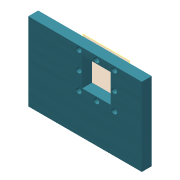
# Autodesk Inventor part: cellSTORM_Base_v0
Saved by Autodesk Inventor 2019 (Build 230136000, 136)
## iProperties
Created: 2019-10-29
Part Number: cellSTORM_Base_v0
Material: Generic
Document SubType Name: Modeling
Designer: diederichbenedict
Density: 1 g/cm^3
Appearance: Cadet Blue
Author: diederichbenedict
Autodesk Inventor part; units mm, degrees
ref_plane "YZ Plane" through (0, 0, 0) normal (1, 0, 0) x (0, 1, 0)
ref_plane "XZ Plane" through (0, 0, 0) normal (0, 1, 0) x (-1, 0, 0)
ref_plane "XY Plane" through (0, 0, 0) normal (0, 0, 1) x (1, 0, 0)
ref_plane "Work Plane1" through (0, 0, 0) normal (0, 0, 1) x (1, 0, 0)
sketch "Sketch1" plane through (0, 0, 0) normal (0, 0, 1) x (1, 0, 0)
  circle A0 centre (0, 25) radius 1.95 construction
  circle A1 centre (-25, 0) radius 1.95 construction
  circle A2 centre (-25, -25) radius 1.95 construction
  circle A3 centre (25, 25) radius 1.95 construction
  circle A4 centre (25, -25) radius 1.95 construction
  circle A5 centre (-25, 25) radius 1.95 construction
  circle A6 centre (25, 0) radius 1.95 construction
  circle A7 centre (0, -25) radius 1.95 construction
  line L0 (-28, 30) -> (-30, 28) construction
  line L1 (-30, 28) -> (-30, -28) construction
  line L2 (-30, -28) -> (-28, -30) construction
  line L3 (-28, -30) -> (28, -30) construction
  line L4 (28, -30) -> (30, -28) construction
  line L5 (30, -28) -> (30, 28) construction
  line L6 (30, 28) -> (28, 30) construction
  line L7 (28, 30) -> (-28, 30) construction
  circle A8 centre (35, -56) radius 1 construction
  circle A9 centre (5, -48.5) radius 1 construction
  circle A10 centre (5, -64.5) radius 1.0474 construction
  circle A11 centre (-5, -64.5) radius 1 construction
  circle A12 centre (-5, -56) radius 1 construction
  circle A13 centre (-5, -48.5) radius 1 construction
  circle A14 centre (5, -56) radius 1 construction
  circle A15 centre (35, -48) radius 1 construction
  circle A16 centre (35, -64) radius 1 construction
  line L8 (38, -40) -> (38, -72) construction
  line L9 (38, -40) -> (-10, -40) construction
  line L10 (-10, -72) -> (-10, -40) construction
  line L11 (38, -72) -> (-10, -72) construction
  line L12 (38, -71) -> (38, -41) construction
  line L13 (38, -71) -> (48, -71) construction
  line L14 (48, -41) -> (48, -71) construction
  line L15 (38, -41) -> (48, -41) construction
  line L16 (56, -75) -> (-52.5, -75)
  line L17 (-52.5, -75) -> (-52.5, -30)
  line L18 (-52.5, -30) -> (56, -30)
  line L19 (56, -30) -> (56, -75)
  line L20 (-40, -41.1445) -> (-40, -68) construction
  line L21 (-41, -39.0927) -> (-41, -47.7587) construction
  line L22 (-41, -39.0927) -> (-46.5, -39.0927) construction
  line L23 (-46.5, -47.7587) -> (-46.5, -39.0927) construction
  line L24 (-41, -47.7587) -> (-46.5, -47.7587) construction
  line L25 (-41, -60.5) -> (-41, -64) construction
  line L26 (-41, -60.5) -> (-46.5, -60.5) construction
  line L27 (-46.5, -64) -> (-46.5, -60.5) construction
  line L28 (-41, -64) -> (-46.5, -64) construction
  line L29 (64, 30) -> (-96, 30)
  line L30 (-96, 30) -> (-96, -80)
  line L31 (-96, -80) -> (64, -80)
  line L32 (64, -80) -> (64, 30)
  line L33 (20, -20) -> (-20, -20)
  line L34 (-20, -20) -> (-20, 20)
  line L35 (-20, 20) -> (20, 20)
  line L36 (20, 20) -> (20, -20)
  line L37 (20, -20) -> (-20, 20) construction
  line L38 (-20, -20) -> (20, 20) construction
  line L39 (-52.5, -30) -> (-30, -30)
  line L40 (-30, -30) -> (-30, -25)
  line L41 (-30, -25) -> (-52.5, -25)
  line L42 (-52.5, -25) -> (-52.5, -30)
  point P0 (0, 0)
  dimension "d1" = 3
  dimension "d2" = 8
  dimension "d4" = 6
  dimension "d5" = 160
  dimension "d6" = 110
  dimension "d7" = 8
  dimension "d19" = 40
  dimension "d20" = 40
  dimension "d28" = 5
  dimension "d29" = 0
  constraints: 36 end point, 8 parallel, 4 horizontal, 4 perpendicular, 2 midpoint, 1 point on line
  measures "d1" distance between parallel lines of L11 L16
  measures "d2" distance between parallel lines of L19 L14
  measures "d4" distance between parallel lines of L27 L17
  measures "d5" distance of L31.end L30.end
  measures "d6" distance of L30.end L29.end
  measures "d7" distance between parallel lines of L32 L19
  measures "d19" distance of L34.end L35.end
  measures "d20" distance of L33.end L34.end
  measures "d28" distance of L40.end L39.end
  measures "d29" distance between parallel lines of L18 L3
extrude "Extrusion1" add sketch "Sketch1" along normal blind 10
sketch "Sketch2" plane through (0, 0, 10) normal (0, 0, 1) x (1, 0, 0)
  line L0 (-30, -30) -> (56, -30) projected
  line L1 (56, -30) -> (56, -75) projected
  line L2 (56, -75) -> (-52.5, -75) projected
  line L3 (64, 30) -> (-96, 30) projected
  line L4 (-96, 30) -> (-96, -80) projected
  line L5 (-96, -80) -> (64, -80) projected
  line L6 (64, -80) -> (64, 30) projected
  line L7 (20, -20) -> (20, 20) projected
  line L8 (-20, -20) -> (20, -20)
  line L9 (20, -20) -> (20, 20)
  line L10 (20, 20) -> (-20, 20)
  line L11 (-20, 20) -> (-20, -20)
  line L12 (-20, -20) -> (20, 20) construction
  line L13 (20, -20) -> (-20, 20) construction
  line L14 (-52.5, -25) -> (-30, -25) projected
  line L15 (-30, -25) -> (-30, -30) projected
  line L16 (-52.5, -75) -> (-52.5, -25) projected
  point P0 (0, 0)
  constraints: 12 end point, 2 midpoint, 2 parallel, 1 horizontal, 1 perpendicular
extrude "Extrusion2" add sketch "Sketch2" along normal blind 4 contours L0 L1 L2 L16 L14 L15 | L6 L5 L4 L3
sketch "Sketch3" plane through (0, 0, 14) normal (0, 0, 1) x (1, 0, 0)
  circle A0 centre (0, 25) radius 1.95 construction
  circle A1 centre (-25, 0) radius 1.95 construction
  circle A2 centre (-25, -25) radius 1.95 construction
  circle A3 centre (25, 25) radius 1.95 construction
  circle A4 centre (25, -25) radius 1.95 construction
  circle A5 centre (-25, 25) radius 1.95 construction
  circle A6 centre (25, 0) radius 1.95 construction
  circle A7 centre (0, -25) radius 1.95 construction
  line L0 (-28, 30) -> (-30, 28) construction
  line L1 (-30, 28) -> (-30, -28) construction
  line L2 (-30, -28) -> (-28, -30) construction
  line L3 (-28, -30) -> (28, -30) construction
  line L4 (28, -30) -> (30, -28) construction
  line L5 (30, -28) -> (30, 28) construction
  line L6 (30, 28) -> (28, 30) construction
  line L7 (28, 30) -> (-28, 30) construction
  point P0 (0, 0)
hole "Hole1" at (25, 25, 14) at (0, 25, 14) at (-25, 25, 14) at (-25, 0, 14) at (-25, -25, 14) at (0, -25, 14) at (25, -25, 14) at (25, 0, 14) direction (0, 0, -1) diameter 3.3 end through all counterbore diameter 8 counterbore depth 5
sketch "Sketch4" plane through (0, 0, 0) normal (0, 0, -1) x (-1, 0, 0)
  line L0 (52.5, -75) -> (-56, -75) construction
  line L1 (-56, -75) -> (-56, -30) construction
  line L2 (-56, -30) -> (30, -30) construction
  line L3 (20, 20) -> (20, -20) construction
  line L4 (20, -20) -> (-20, -20) construction
  line L5 (-20, -20) -> (-20, 20) construction
  line L6 (-20, 20) -> (20, 20) construction
  line L7 (-64, 30) -> (96, 30) construction
  line L8 (-64, -80) -> (-64, 30) construction
  line L9 (96, -80) -> (-64, -80) construction
  line L10 (96, 30) -> (96, -80) construction
  line L11 (54.8114, -67.6244) -> (54.8114, -43.3756) construction
  line L12 (54.8114, -43.3756) -> (75.8114, -55.5) construction
  line L13 (75.8114, -55.5) -> (54.8114, -67.6244) construction
  line L14 (96, 30) -> (96, -80) construction
  line L15 (30, -30) -> (30, -25) projected
  line L16 (30, -25) -> (52.5, -25) projected
  line L17 (52.5, -25) -> (52.5, -75) projected
  line L18 (20, -49.5) -> (16.4, -49.5)
  line L19 (20, -61.5) -> (16.4, -61.5)
  circle A0 centre (5, -55.5) radius 1.8 projected
  point P0 (0, 0)
  point P1 (61.8114, -55.5)
  dimension "d30" = 21
  dimension "d31" = 0
  constraints: 10 end point, 2 horizontal, 1 parallel, 11 other
  measures "d30" distance from line of L11 L12.end
  measures "d31" vertical distance of A0.centre point (61.811, -55.5)
hole "Hole2" at (-54.8114, -43.3756, 0) at (-75.8114, -55.5, 0) at (-54.8114, -67.6244, 0) direction (0, 0, 1) diameter 2.8 depth 12 tip angle 118
body "Solid1"
